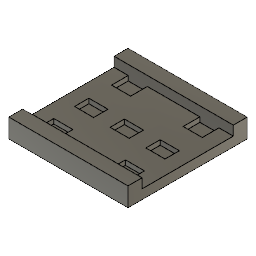
LedDice2 v4 (Autodesk Fusion 360 design; units mm, degrees)
Autodesk Fusion 360 part; units mm, degrees
note: some values were not read from the file. Chosen so that the rebuilt part matches the saved one: which face or edge a step refers to. Set by a fixed rule: which sketch regions a step uses.
sketch "Sketch1" plane through (0, 0, 0) normal (0, 0, 1) x (1, 0, 0)
  line L0 (0, 0) -> (25, 0)
  line L1 (25, 0) -> (25, 25)
  line L2 (25, 25) -> (0, 25)
  line L3 (0, 25) -> (0, 0)
  dimension "d1" = 25
  dimension "d2" = 25
  constraint horizontal L0
  constraint vertical L1
  constraint horizontal L2
  constraint vertical L3
  constraint coincident L0.start L3.end
  measures "d1" distance of L1.end L2.end
  measures "d2" distance of L0.end L1.end
  measures "d5" distance of L0.start
  measures "d6" distance of L0.start
  measures "d10" distance of L0.start
  measures "d12" distance of L0.start
  measures "d20" distance of L0.start
  measures "d46" distance of L0.start
  measures "d47" distance of L0.start
extrude "Extrude1" add sketch "Sketch1" along normal blind 1
sketch "Sketch2" plane through (0, 0, 1) normal (0, 0, 1) x (-1, 0, 0)
  line L0 (0, -25) -> (0, 0)
  line L1 (0, 0) -> (-25, 0)
  line L2 (-25, 0) -> (-25, -25)
  line L3 (-25, -25) -> (0, -25)
  line L4 (0, -22.05) -> (-23, -22.05)
  line L5 (-23, -22.05) -> (-23, -2.95)
  line L6 (-23, -2.95) -> (0, -2.95)
  line L7 (0, -2.95) -> (0, -22.05)
  dimension "d5" = 19.1
  dimension "d6" = 2.95
  constraint horizontal L4
  constraint vertical L5
  constraint horizontal L6
  constraint vertical L7
  constraint coincident L0 L4.start
  measures "d5" distance of L4.end L5.end
  measures "d6" distance of L3 L4
extrude "Extrude2" add sketch "Sketch2" along normal blind 3 contours L0 L1 L2 L3 L4 L5 L6
sketch "Sketch3" plane through (0, 0, 1) normal (0, 0, 1) x (-1, 0, 0)
  line L0 (-23, -22.05) -> (0, -22.05)
  line L1 (0, -22.05) -> (0, -2.95)
  line L2 (0, -2.95) -> (-23, -2.95)
  line L3 (-23, -2.95) -> (-23, -22.05)
  line L4 (-16.5, -22.05) -> (-20.5, -22.05)
  line L5 (-20.5, -22.05) -> (-20.5, -18.55)
  line L6 (-20.5, -18.55) -> (-16.5, -18.55)
  line L7 (-16.5, -18.55) -> (-16.5, -22.05)
  line L8 (-5.5, -18.55) -> (-1.5, -18.55)
  line L9 (-5.5, -22.05) -> (-5.5, -18.55)
  line L10 (-1.5, -18.55) -> (-1.5, -22.05)
  line L11 (-1.5, -22.05) -> (-5.5, -22.05)
  line L12 (-20.5, -2.95) -> (-16.5, -2.95)
  line L13 (-20.5, -6.45) -> (-20.5, -2.95)
  line L14 (-16.5, -2.95) -> (-16.5, -6.45)
  line L15 (-16.5, -6.45) -> (-20.5, -6.45)
  line L16 (-5.5, -2.95) -> (-1.5, -2.95)
  line L17 (-5.5, -6.45) -> (-5.5, -2.95)
  line L18 (-1.5, -2.95) -> (-1.5, -6.45)
  line L19 (-1.5, -6.45) -> (-5.5, -6.45)
  line L20 (-9, -13.75) -> (-13, -13.75)
  line L21 (-13, -13.75) -> (-13, -10.75)
  line L22 (-13, -10.75) -> (-9, -10.75)
  line L23 (-9, -10.75) -> (-9, -13.75)
  line L24 (-16.4916, -13.75) -> (-20.4916, -13.75)
  line L25 (-20.4916, -13.75) -> (-20.4916, -10.75)
  line L26 (-20.4916, -10.75) -> (-16.4916, -10.75)
  line L27 (-16.4916, -10.75) -> (-16.4916, -13.75)
  line L28 (-5.5, -13.7991) -> (-1.5, -13.7991)
  line L29 (-1.5, -13.7991) -> (-1.5, -10.7991)
  line L30 (-1.5, -10.7991) -> (-5.5, -10.7991)
  line L31 (-5.5, -10.7991) -> (-5.5, -13.7991)
  dimension "d10" = 3.5
  dimension "d11" = 4
  dimension "d12" = 2.5
  dimension "d16" = 15
  dimension "d17" = 15.6
  dimension "d18" = 4
  dimension "d19" = 3
  dimension "d20" = 3.5
  dimension "d21" = 4.8
  dimension "d50" = 4
  dimension "d51" = 3
  dimension "d52" = 3
  dimension "d53" = 4
  constraint horizontal L4
  constraint vertical L5
  constraint horizontal L6
  constraint vertical L7
  constraint coincident L0.start L4
  constraint horizontal L20
  constraint vertical L21
  constraint horizontal L22
  constraint vertical L23
  constraint horizontal L24
  constraint vertical L25
  constraint horizontal L26
  constraint vertical L27
  constraint horizontal L28
  constraint vertical L29
  constraint horizontal L30
  constraint vertical L31
  measures "d10" distance of L4.end L5.end
  measures "d11" distance of L5.end L6.end
  measures "d12" distance of L3 L5
  measures "d18" distance of L20.start L20.end
  measures "d19" distance of L20.end L21.end
  measures "d20" distance of L7 L21
  measures "d21" distance of L6 L20
  measures "d50" distance of L24.start L24.end
  measures "d51" distance of L24.start L26.end
  measures "d52" distance of L28.end L29.end
  measures "d53" distance of L29.end L30.end
extrude "Extrude3" add sketch "Sketch3" along normal blind 1 contours L0 L1 L2 L3 L5 L6 L7 L8 L9 L10 L13 L14 L15 L17 L18 L19
sketch "Sketch4" plane through (0, 0, 4) normal (0, 0, 1) x (-1, 0, 0)
  line L0 (-23, -2.95) -> (0, -2.95)
  line L1 (0, -2.95) -> (0, 0)
  line L2 (0, 0) -> (-25, 0)
  line L3 (-25, 0) -> (-25, -25)
  line L4 (-25, -25) -> (0, -25)
  line L5 (0, -25) -> (0, -22.05)
  line L6 (0, -22.05) -> (-23, -22.05)
  line L7 (-23, -22.05) -> (-23, -2.95)
  line L8 (-5.5, -18.55) -> (-5.5, -22.05)
  line L9 (-5.5, -22.05) -> (-1.5, -22.05)
  line L10 (-1.5, -22.05) -> (-1.5, -18.55)
  line L11 (-1.5, -18.55) -> (-5.5, -18.55)
  line L12 (-16.5, -22.05) -> (-16.5, -18.55)
  line L13 (-16.5, -18.55) -> (-20.5, -18.55)
  line L14 (-20.5, -18.55) -> (-20.5, -22.05)
  line L15 (-20.5, -22.05) -> (-16.5, -22.05)
  line L16 (-1.5, -6.45) -> (-1.5, -2.95)
  line L17 (-1.5, -2.95) -> (-5.5, -2.95)
  line L18 (-5.5, -2.95) -> (-5.5, -6.45)
  line L19 (-5.5, -6.45) -> (-1.5, -6.45)
  line L20 (-20.5, -2.95) -> (-20.5, -6.45)
  line L21 (-20.5, -6.45) -> (-16.5, -6.45)
  line L22 (-16.5, -6.45) -> (-16.5, -2.95)
  line L23 (-16.5, -2.95) -> (-20.5, -2.95)
  line L24 (-2, -25) -> (-5.5, -25)
  line L25 (-5.5, -25) -> (-5.5, -21)
  line L26 (-5.5, -21) -> (-2, -21)
  line L27 (-2, -21) -> (-2, -25)
  line L28 (-17, -25) -> (-20.5, -25)
  line L29 (-20.5, -25) -> (-20.5, -21)
  line L30 (-20.5, -21) -> (-17, -21)
  line L31 (-17, -21) -> (-17, -25)
  line L32 (-2, 0) -> (-5.5, 0)
  line L33 (-5.5, 0) -> (-5.5, -4)
  line L34 (-5.5, -4) -> (-2, -4)
  line L35 (-2, -4) -> (-2, 0)
  line L36 (-17, 0) -> (-20.5, 0)
  line L37 (-20.5, 0) -> (-20.5, -4)
  line L38 (-20.5, -4) -> (-17, -4)
  line L39 (-17, -4) -> (-17, 0)
  dimension "d24" = 4
  dimension "d25" = 4
  dimension "d26" = 4
  dimension "d27" = 4
  constraint horizontal L24
  constraint vertical L25
  constraint horizontal L26
  constraint vertical L27
  constraint coincident L8 L25.end
  constraint coincident L4 L24.start
  constraint horizontal L28
  constraint vertical L29
  constraint horizontal L30
  constraint vertical L31
  constraint coincident L14 L29.end
  constraint coincident L4 L28.start
  constraint horizontal L32
  constraint vertical L33
  constraint horizontal L34
  constraint vertical L35
  constraint coincident L18 L33.end
  constraint coincident L2 L32.start
  constraint horizontal L36
  constraint vertical L37
  constraint horizontal L38
  constraint vertical L39
  constraint coincident L20 L37.end
  constraint coincident L2 L36.start
  measures "d24" distance of L24 L26
  measures "d25" distance of L28 L30
  measures "d26" distance of L36 L38
  measures "d27" distance of L32 L34
extrude "Extrude4" add sketch "Sketch4" along normal blind 2 contours L0 L2 L3 L4 L6 L7 L29 L37 | L0 L2 L23 L36 L37 L39 | L0 L20 L23 L37 L38 L39 | L0 L2 L23 L33 L39 | L6 L14 L15 L29 L30 L31 | L4 L6 L15 L28 L29 L31 | L4 L6 L15 L25 L31 | L0 L2 L17 L32 L33 L35 | L0 L17 L18 L33 L34 L35 | L0 L1 L2 L17 L35 | L6 L8 L9 L25 L26 L27 | L4 L6 L9 L24 L25 L27 | L4 L5 L6 L9 L27
chamfer "Chamfer2" distance 0.6 angle 60 2 edges at (18.75, 4, 4) (3.75, 4, 4) measured on face at (19.3333, 4, 4.6667) measured on face at (4.3333, 4, 4.6667)
chamfer "Chamfer1" distance 1 angle 30 2 edges at (3.75, 21, 4) (18.75, 21, 4) measured on face at (4.3333, 21.35, 4) measured on face at (18.1667, 21.7, 4)
chamfer "Chamfer5" distance 1 angle 45 4 edges at (3.75, 21, 6) (18.75, 21, 6) (18.75, 4, 6) (3.75, 4, 6) measured on face at (14, 24.0167, 6) measured on face at (14, 24.0167, 6) measured on face at (14, 24.0167, 6) measured on face at (14, 24.0167, 6)
sketch "Sketch6" plane through (0, 0, 0) normal (-1, 0, 0) x (0, -1, 0)
  line L0 (-25, 0) -> (0, 0)
  line L1 (0, 0) -> (0, 6)
  line L2 (0, 6) -> (-2.95, 6)
  line L3 (-2.95, 6) -> (-2.95, 2)
  line L4 (-2.95, 2) -> (-22.05, 2)
  line L5 (-22.05, 2) -> (-22.05, 6)
  line L6 (-22.05, 6) -> (-25, 6)
  line L7 (-25, 6) -> (-25, 0)
  line L8 (-21.25, 6) -> (-3.75, 6)
  line L9 (-3.75, 6) -> (-3.75, 3.5)
  line L10 (-3.75, 3.5) -> (-21.25, 3.5)
  line L11 (-21.25, 3.5) -> (-21.25, 6)
  dimension "d46" = 17.5
  dimension "d47" = 3.75
  constraint horizontal L8
  constraint vertical L9
  constraint horizontal L10
  constraint vertical L11
  measures "d46" distance of L9.end L10.end
  measures "d47" distance of L7 L11
extrude "Extrude6" cut sketch "Sketch6" against normal blind 22.5 contours L8 L9 L10 L11
sketch "Sketch7" plane through (0, 0, 6) normal (0, 0, 1) x (-1, 0, 0)
  line L0 (-5.5, -3) -> (-2, -3)
  line L1 (-2, -3) -> (-2, -2.95)
  line L2 (-2, -2.95) -> (0, -2.95)
  line L3 (0, -2.95) -> (0, 0)
  line L4 (0, 0) -> (-25, 0)
  line L5 (-25, 0) -> (-25, -25)
  line L6 (-25, -25) -> (0, -25)
  line L7 (0, -25) -> (0, -22.05)
  line L8 (0, -22.05) -> (-2, -22.05)
  line L9 (-2, -22.05) -> (-2, -22)
  line L10 (-2, -22) -> (-5.5, -22)
  line L11 (-5.5, -22) -> (-5.5, -22.05)
  line L12 (-5.5, -22.05) -> (-17, -22.05)
  line L13 (-17, -22.05) -> (-17, -22)
  line L14 (-17, -22) -> (-20.5, -22)
  line L15 (-20.5, -22) -> (-20.5, -22.05)
  line L16 (-20.5, -22.05) -> (-23, -22.05)
  line L17 (-23, -22.05) -> (-23, -2.95)
  line L18 (-23, -2.95) -> (-20.5, -2.95)
  line L19 (-20.5, -2.95) -> (-20.5, -3)
  line L20 (-20.5, -3) -> (-17, -3)
  line L21 (-17, -3) -> (-17, -2.95)
  line L22 (-17, -2.95) -> (-5.5, -2.95)
  line L23 (-5.5, -2.95) -> (-5.5, -3)
  line L24 (-25, -25) -> (-23, -25)
  line L25 (-23, -25) -> (-23, 0)
  line L26 (-23, 0) -> (-25, 0)
  line L27 (-25, 0) -> (-25, -25)
  constraint horizontal L24
  constraint vertical L25
  constraint horizontal L26
  constraint vertical L27
  constraint coincident L4 L25.end
  constraint coincident L5.end L6.start
extrude "Extrude7" cut sketch "Sketch7" against normal blind 6 contours L4 L5 L6 L17 L24 L25 L26 L27
sketch "Sketch8" plane through (0, 0, 0) normal (-1, 0, 0) x (0, -1, 0)
  line L0 (-25, 0) -> (0, 0)
  line L1 (0, 0) -> (0, 6)
  line L2 (0, 6) -> (-2.95, 6)
  line L3 (-2.95, 6) -> (-2.95, 2)
  line L4 (-2.95, 2) -> (-22.05, 2)
  line L5 (-22.05, 2) -> (-22.05, 6)
  line L6 (-22.05, 6) -> (-25, 6)
  line L7 (-25, 6) -> (-25, 0)
extrude "Extrude8" add sketch "Sketch8" along normal blind 1.5
sketch "Sketch9" plane through (23, 0, 0) normal (1, 0, 0) x (0, 1, 0)
  line L0 (2.95, 2) -> (2.95, 6)
  line L1 (2.95, 6) -> (0, 6)
  line L2 (0, 6) -> (0, 0)
  line L3 (0, 0) -> (25, 0)
  line L4 (25, 0) -> (25, 6)
  line L5 (25, 6) -> (22.05, 6)
  line L6 (22.05, 6) -> (22.05, 2)
  line L7 (22.05, 2) -> (2.95, 2)
extrude "Extrude9" add sketch "Sketch9" along normal blind 0.5
sketch "Sketch11" plane through (0, 0, 6) normal (0, 0, 1) x (-1, 0, 0)
  line L0 (-23.5, -2.95) -> (-20.5, -2.95)
  line L1 (-20.5, -2.95) -> (-20.5, -3)
  line L2 (-20.5, -3) -> (-17, -3)
  line L3 (-17, -3) -> (-17, -2.95)
  line L4 (-17, -2.95) -> (-5.5, -2.95)
  line L5 (-5.5, -2.95) -> (-5.5, -3)
  line L6 (-5.5, -3) -> (-2, -3)
  line L7 (-2, -3) -> (-2, -2.95)
  line L8 (-2, -2.95) -> (1.5, -2.95)
  line L9 (1.5, -2.95) -> (1.5, 0)
  line L10 (1.5, 0) -> (-23.5, 0)
  line L11 (-23.5, 0) -> (-23.5, -2.95)
  line L12 (2, -25) -> (-23.5, -25)
  line L13 (-23.5, -25) -> (-23.5, 0)
  line L14 (-23.5, 0) -> (2, 0)
  line L15 (2, 0) -> (2, -25)
  constraint horizontal L12
  constraint vertical L13
  constraint horizontal L14
  constraint vertical L15
  constraint coincident L10.end L11.start
extrude "Extrude10" cut sketch "Sketch11" against normal blind 2
sketch "Sketch10" plane through (0, 0, 6) normal (0, 0, 1) x (-1, 0, 0)
  line L0 (-23.5, -25) -> (1.5, -25)
  line L1 (1.5, -25) -> (1.5, -22.05)
  line L2 (1.5, -22.05) -> (-2, -22.05)
  line L3 (-2, -22.05) -> (-2, -22)
  line L4 (-2, -22) -> (-5.5, -22)
  line L5 (-5.5, -22) -> (-5.5, -22.05)
  line L6 (-5.5, -22.05) -> (-17, -22.05)
  line L7 (-17, -22.05) -> (-17, -22)
  line L8 (-17, -22) -> (-20.5, -22)
  line L9 (-20.5, -22) -> (-20.5, -22.05)
  line L10 (-20.5, -22.05) -> (-23.5, -22.05)
  line L11 (-23.5, -22.05) -> (-23.5, -25)
  line L12 (-2, -22) -> (-1.8, -22)
  line L13 (-1.8, -22) -> (-1.8, -25)
  line L14 (-1.8, -25) -> (-2, -25)
  line L15 (-2, -25) -> (-2, -22)
  line L16 (-5.5, -22) -> (-5.7, -22)
  line L17 (-5.7, -22) -> (-5.7, -25)
  line L18 (-5.7, -25) -> (-5.5, -25)
  line L19 (-5.5, -25) -> (-5.5, -22)
  line L20 (-17, -22) -> (-16.8, -22)
  line L21 (-16.8, -22) -> (-16.8, -25)
  line L22 (-16.8, -25) -> (-17, -25)
  line L23 (-17, -25) -> (-17, -22)
  line L24 (-20.5, -22) -> (-20.7, -22)
  line L25 (-20.7, -22) -> (-20.7, -25.4)
  line L26 (-20.7, -25.4) -> (-20.5, -25.4)
  line L27 (-20.5, -25.4) -> (-20.5, -22)
  line L28 (-2, -3) -> (-1.8, -3)
  line L29 (-1.8, -3) -> (-1.8, 0)
  line L30 (-1.8, 0) -> (-2, 0)
  line L31 (-2, 0) -> (-2, -3)
  line L32 (-5.5, 0) -> (-5.6867, 0)
  line L33 (-5.6867, 0) -> (-5.6867, -3)
  line L34 (-5.6867, -3) -> (-5.5, -3)
  line L35 (-5.5, -3) -> (-5.5, 0)
  dimension "d60" = 0.2
  dimension "d61" = 0.2
  dimension "d62" = 0.2
  dimension "d63" = 0.2
  constraint horizontal L12
  constraint vertical L13
  constraint horizontal L14
  constraint vertical L15
  constraint coincident L0 L13.end
  constraint coincident L3.end L4.start
  constraint horizontal L16
  constraint vertical L17
  constraint horizontal L18
  constraint vertical L19
  constraint coincident L0 L17.end
  constraint coincident L4.end L5.start
  constraint horizontal L20
  constraint vertical L21
  constraint horizontal L22
  constraint vertical L23
  constraint coincident L0 L21.end
  constraint coincident L7.end L8.start
  constraint horizontal L24
  constraint vertical L25
  constraint horizontal L26
  constraint vertical L27
  constraint coincident L8.end L9.start
  constraint horizontal L28
  constraint vertical L29
  constraint horizontal L30
  constraint vertical L31
  constraint horizontal L32
  constraint vertical L33
  constraint horizontal L34
  constraint vertical L35
  measures "d60" distance of L13.end L14.end
  measures "d61" distance of L21.end L22.end
  measures "d62" distance of L17.end L18.end
  measures "d63" distance of L25.end L26.end
equation "d6 = ( d1 - d5 ) / 2"
equation "d17 = 16.10 mm - 0.5 mm"
equation "d21 = 5.05 mm - 0.25 mm"
